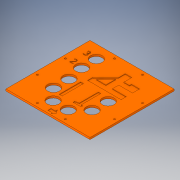
# Autodesk Inventor part: ControlPlateClimber
Saved by Autodesk Inventor 2019 (Build 230136000, 136)
## iProperties
Created: 2019-01-04
Part Number: ControlPlateClimber
Material: Generic
Document SubType Name: Modeling
Designer: james
Density: 1 g/cm^3
Appearance: Default(1)
Author: james
Autodesk Inventor part; units mm, degrees
ref_plane "YZ Plane" through (0, 0, 0) normal (1, 0, 0) x (0, 1, 0)
ref_plane "XZ Plane" through (0, 0, 0) normal (0, 1, 0) x (-1, 0, 0)
ref_plane "XY Plane" through (0, 0, 0) normal (0, 0, 1) x (1, 0, 0)
sketch "Sketch1" plane through (0, 0, 0) normal (0, 1, 0) x (-1, 0, 0)
  line L0 (148.429, 108.1825) -> (-80.171, 108.1825)
  line L1 (-80.171, 108.1825) -> (-80.171, -120.4175)
  line L2 (-80.171, -120.4175) -> (148.429, -120.4175)
  line L3 (148.429, -120.4175) -> (148.429, 108.1825)
  point P0 (0, 0)
  dimension "d0" = 228.6
  dimension "d1" = 228.6
  constraints: 8 end point, 2 parallel, 1 horizontal, 1 perpendicular
  measures "d0" distance of L0.end L1.end
  measures "d1" distance of L0.start L0.end
extrude "Extrusion1" add sketch "Sketch1" along normal blind 5.08
sketch "Sketch2" plane through (0, 5.08, 0) normal (0, 1, 0) x (1, 0, 0)
  line L0 (-148.429, -108.1825) -> (80.171, -108.1825) projected
  line L1 (80.171, 120.4175) -> (-148.429, 120.4175) projected
  line L2 (-148.429, 120.4175) -> (-148.429, -108.1825) projected
  line L3 (80.171, -108.1825) -> (80.171, 120.4175) projected
  point P0 (0, 0)
  point P1 (-138.904, -31.9825)
  point P2 (-138.904, 44.2175)
  point P3 (-72.229, 110.8925)
  point P4 (3.971, 110.8925)
  point P5 (70.646, 44.2175)
  point P6 (70.646, -31.9825)
  point P7 (-72.229, -98.6575)
  point P8 (3.971, -98.6575)
  dimension "d4" = 76.2
  dimension "d5" = 76.2
  dimension "d6" = 76.2
  dimension "d7" = 9.525
  dimension "d8" = 9.525
  dimension "d9" = 76.2
  dimension "d10" = 9.525
  dimension "d11" = 76.2
  dimension "d12" = 9.525
  dimension "d13" = 9.525
  measures "d4" distance from line of L0 point (-138.904, -31.983)
  measures "d5" distance of point (-138.904, 44.217) point (-138.904, -31.983)
  measures "d6" distance from line of L1 point (-138.904, 44.217)
  measures "d7" distance from line of L2 point (-138.904, 44.217)
  measures "d8" distance from line of L2 point (-138.904, -31.983)
  measures "d9" distance from line of point (-72.229, 110.892) L2
  measures "d10" distance from line of L1 point (-72.229, 110.892)
  measures "d11" distance of point (3.971, 110.892) point (-72.229, 110.892)
  measures "d12" distance from line of L3 point (70.646, 44.217)
  measures "d13" distance from line of L0 point (-72.229, -98.658)
hole "Hole1" at (-138.904, 5.08, 31.9825) at (-138.904, 5.08, -44.2175) at (-72.229, 5.08, -110.8925) at (3.971, 5.08, -110.8925) at (70.646, 5.08, -44.2175) at (70.646, 5.08, 31.9825) at (-72.229, 5.08, 98.6575) at (3.971, 5.08, 98.6575) direction (0, -1, 0) diameter 4.826 end through all
sketch "Sketch4" plane through (0, 5.08, 0) normal (0, 1, 0) x (1, 0, 0)
  line L0 (-57.5475, 37.222) -> (33.43, 37.222)
  line L1 (33.43, 37.222) -> (33.43, 23.0153)
  line L2 (33.43, 23.0153) -> (-57.5475, 23.0153)
  line L3 (-57.5475, 23.0153) -> (-57.5475, 37.222)
  line L4 (-22.0308, 37.222) -> (-3.9992, 37.222)
  line L5 (-3.9992, 37.222) -> (-3.9992, 89.9507)
  line L6 (-3.9992, 89.9507) -> (-22.0308, 89.9507)
  line L7 (-22.0308, 89.9507) -> (-22.0308, 37.222)
  line L8 (-22.0308, 71.0995) -> (-55.0887, 37.222)
  line L9 (-22.0308, 63.5863) -> (-47.7573, 37.222)
  line L10 (11.3003, 73.5584) -> (33.43, 73.5584)
  line L11 (33.43, 73.5584) -> (33.43, 54.1607)
  line L12 (33.43, 54.1607) -> (11.3003, 54.1607)
  line L13 (11.3003, 54.1607) -> (11.3003, 73.5584)
  line L14 (11.3003, 54.1607) -> (-3.9992, 54.1607)
  line L15 (11.3003, 68.0942) -> (-3.9992, 68.0942)
  point P0 (0, 0)
  constraints: 32 end point, 7 parallel, 7 point on line, 4 perpendicular, 3 horizontal, 1 midpoint
extrude "Extrusion2" cut sketch "Sketch4" against normal blind 1.651 contours L0 L1 L2 L3 | L8 L7 L9 L0 | L7 L6 L5 L0 | L5 L15 L13 L14 | L13 L10 L11 L12
sketch "Sketch5" plane through (0, 5.08, 0) normal (0, 1, 0) x (1, 0, 0)
  point P0 (0, 0)
  point P1 (-96.0634, 85.1626)
  point P2 (-95.5184, 44.5571)
  point P3 (19.7577, 1.7714)
  point P4 (18.6676, -41.0143)
  point P5 (-86.5252, 1.2263)
  point P6 (-86.5252, -40.7418)
  point P7 (-14.5798, -72.6266)
  point P8 (-56.8205, -71.5366)
hole "Hole2" at (-96.0634, 5.08, -85.1626) at (-95.5184, 5.08, -44.5571) at (19.7577, 5.08, -1.7714) at (18.6676, 5.08, 41.0143) at (-86.5252, 5.08, -1.2263) at (-86.5252, 5.08, 40.7418) at (-14.5798, 5.08, 72.6266) at (-56.8205, 5.08, 71.5366) direction (0, -1, 0) diameter 31.75 depth 25.4 tip angle 118.188
sketch "Sketch6" plane through (0, 5.08, 0) normal (0, 1, 0) x (1, 0, 0)
  line L0 (-63.361, 9.947) -> (-63.361, -48.3723)
  line L1 (-63.361, -48.3723) -> (-55.4579, -48.3723)
  line L2 (-55.4579, -48.3723) -> (-55.4579, 9.947)
  line L3 (-55.4579, 9.947) -> (-63.361, 9.947)
  line L4 (-15.3974, 9.947) -> (-8.5844, 9.947)
  line L5 (-8.5844, 9.947) -> (-8.5844, -43.467)
  line L6 (-8.5844, -43.467) -> (-3.9515, -43.467)
  line L7 (-3.9515, -43.467) -> (-3.9515, -48.3723)
  line L8 (-3.9515, -48.3723) -> (-25.7532, -48.3723)
  line L9 (-25.7532, -48.3723) -> (-25.7532, -43.467)
  line L10 (-25.7532, -43.467) -> (-15.3974, -42.1044)
  line L11 (-15.3974, -42.1044) -> (-15.3974, 9.947)
  line L12 (-41.1372, -92.7706) -> (-29.2067, -92.7706)
  line L13 (-29.2067, -92.7706) -> (-29.2067, -87.6575)
  line L14 (-29.2067, -87.6575) -> (-21.9024, -97.8836)
  line L15 (-21.9024, -97.8836) -> (-29.2067, -104.9445)
  line L16 (-29.2067, -104.9445) -> (-29.2067, -101.4141)
  line L17 (-29.2067, -101.4141) -> (-41.1372, -101.4141)
  line L18 (-41.1372, -101.4141) -> (-41.1372, -92.7706)
  point P0 (0, 0)
  constraints: 38 end point, 10 perpendicular, 7 point on line, 1 horizontal, 1 parallel, 1 vertical
extrude "Extrusion3" cut sketch "Sketch6" against normal blind 1.651
sketch "Sketch7" plane through (0, 5.08, 0) normal (0, 1, 0) x (1, 0, 0)
  line L0 (-127.4032, 94.1557) -> (-105.6016, 94.1557) construction
  line L1 (-105.6016, 94.1557) -> (-105.6016, 63.361) construction
  line L2 (-105.6016, 63.361) -> (-127.4032, 63.361) construction
  line L3 (-127.4032, 63.361) -> (-127.4032, 94.1557) construction
  spline S0 degree 2 poles (-122.1791, 92.3897) (-122.7349, 92.3897) (-123.834, 92.118) (-124.3651, 91.908) knots 0 0 0 1 2 2 2
  spline S1 degree 2 poles (-124.3651, 91.908) (-124.8591, 91.6981) (-125.5878, 91.2535) (-125.8718, 91.0559) knots 0 0 0 1 2 2 2
  line L4 (-125.8718, 91.0559) -> (-125.9953, 91.0559)
  line L5 (-125.9953, 91.0559) -> (-125.9953, 93.2171)
  spline S2 degree 2 poles (-125.9953, 93.2171) (-125.3284, 93.5753) (-123.0436, 94.1557) (-122.0186, 94.1557) knots 0 0 0 1 2 2 2
  spline S3 degree 2 poles (-122.0186, 94.1557) (-120.9812, 94.1557) (-119.4374, 93.7358) (-118.8076, 93.2912) knots 0 0 0 1 2 2 2
  spline S4 degree 2 poles (-118.8076, 93.2912) (-118.1407, 92.8096) (-117.4491, 91.414) (-117.4491, 90.4754) knots 0 0 0 1 2 2 2
  spline S5 degree 2 poles (-117.4491, 90.4754) (-117.4491, 89.2157) (-119.104, 87.3138) (-120.2649, 87.0668) knots 0 0 0 1 2 2 2
  line L6 (-120.2649, 87.0668) -> (-120.2649, 86.9186)
  spline S6 degree 2 poles (-120.2649, 86.9186) (-119.7832, 86.8198) (-118.6841, 86.3752) (-118.2148, 85.9306) knots 0 0 0 1 2 2 2
  spline S7 degree 2 poles (-118.2148, 85.9306) (-117.7455, 85.4983) (-117.1527, 84.1151) (-117.1527, 83.1148) knots 0 0 0 1 2 2 2
  spline S8 degree 2 poles (-117.1527, 83.1148) (-117.1527, 82.0897) (-117.8566, 80.3484) (-118.4988, 79.6815) knots 0 0 0 1 2 2 2
  spline S9 degree 2 poles (-118.4988, 79.6815) (-119.1657, 78.9898) (-121.0553, 78.2735) (-122.2532, 78.2735) knots 0 0 0 1 2 2 2
  spline S10 degree 2 poles (-122.2532, 78.2735) (-123.4018, 78.2735) (-125.6495, 78.8293) (-126.4152, 79.2121) knots 0 0 0 1 2 2 2
  line L7 (-126.4152, 79.2121) -> (-126.4152, 81.3734)
  line L8 (-126.4152, 81.3734) -> (-126.267, 81.3734)
  spline S11 degree 2 poles (-126.267, 81.3734) (-125.6248, 80.9041) (-123.4512, 80.0396) (-122.3767, 80.0396) knots 0 0 0 1 2 2 2
  spline S12 degree 2 poles (-122.3767, 80.0396) (-121.7469, 80.0396) (-120.4872, 80.4348) (-120.0673, 80.8918) knots 0 0 0 1 2 2 2
  spline S13 degree 2 poles (-120.0673, 80.8918) (-119.6597, 81.3487) (-119.2275, 82.4355) (-119.2275, 83.263) knots 0 0 0 1 2 2 2
  spline S14 degree 2 poles (-119.2275, 83.263) (-119.2275, 84.0904) (-119.7091, 85.1649) (-120.1414, 85.4736) knots 0 0 0 1 2 2 2
  spline S15 degree 2 poles (-120.1414, 85.4736) (-120.5736, 85.7824) (-121.7469, 86.017) (-122.4385, 86.017) knots 0 0 0 1 2 2 2
  line L9 (-122.4385, 86.017) -> (-123.303, 86.017)
  line L10 (-123.303, 86.017) -> (-123.303, 87.709)
  line L11 (-123.303, 87.709) -> (-122.6237, 87.709)
  spline S16 degree 2 poles (-122.6237, 87.709) (-121.2529, 87.709) (-119.5239, 89.0181) (-119.5239, 90.2655) knots 0 0 0 1 2 2 2
  spline S17 degree 2 poles (-119.5239, 90.2655) (-119.5239, 90.8459) (-119.9685, 91.6734) (-120.3266, 91.9204) knots 0 0 0 1 2 2 2
  spline S18 degree 2 poles (-120.3266, 91.9204) (-120.7095, 92.1797) (-121.6481, 92.3897) (-122.1791, 92.3897) knots 0 0 0 1 2 2 2
  point P0 (0, 0)
  constraints: 2 other
extrude "Extrusion4" cut sketch "Sketch7" against normal blind 1.651
sketch "Sketch8" plane through (0, 5.08, 0) normal (0, 1, 0) x (1, 0, 0)
  line L0 (-127.2171, 57.5261) -> (-116.4954, 57.5261) construction
  line L1 (-116.4954, 57.5261) -> (-116.4954, 35.2579) construction
  line L2 (-116.4954, 35.2579) -> (-127.2171, 35.2579) construction
  line L3 (-127.2171, 35.2579) -> (-127.2171, 57.5261) construction
  line L4 (-116.7072, 41.965) -> (-126.1056, 41.965)
  line L5 (-126.1056, 41.965) -> (-126.1056, 44.1262)
  spline S0 degree 2 poles (-126.1056, 44.1262) (-125.0929, 45.0772) (-123.2898, 46.8432) (-122.4253, 47.7942) knots 0 0 0 1 2 2 2
  spline S1 degree 2 poles (-122.4253, 47.7942) (-120.6839, 49.7085) (-119.4119, 52.0056) (-119.4119, 53.2282) knots 0 0 0 1 2 2 2
  spline S2 degree 2 poles (-119.4119, 53.2282) (-119.4119, 53.8704) (-119.8071, 54.8337) (-120.1652, 55.1425) knots 0 0 0 1 2 2 2
  spline S3 degree 2 poles (-120.1652, 55.1425) (-120.5234, 55.4512) (-121.462, 55.76) (-122.0301, 55.76) knots 0 0 0 1 2 2 2
  spline S4 degree 2 poles (-122.0301, 55.76) (-122.5735, 55.76) (-123.685, 55.4883) (-124.1913, 55.2783) knots 0 0 0 1 2 2 2
  spline S5 degree 2 poles (-124.1913, 55.2783) (-124.6236, 55.1054) (-125.4264, 54.6114) (-125.6734, 54.4385) knots 0 0 0 1 2 2 2
  line L6 (-125.6734, 54.4385) -> (-125.7845, 54.4385)
  line L7 (-125.7845, 54.4385) -> (-125.7845, 56.6122)
  spline S6 degree 2 poles (-125.7845, 56.6122) (-125.1547, 56.9209) (-122.8946, 57.5261) (-121.8819, 57.5261) knots 0 0 0 1 2 2 2
  spline S7 degree 2 poles (-121.8819, 57.5261) (-119.7453, 57.5261) (-117.3371, 55.266) (-117.3371, 53.3394) knots 0 0 0 1 2 2 2
  spline S8 degree 2 poles (-117.3371, 53.3394) (-117.3371, 52.4378) (-117.757, 50.9311) (-118.1275, 50.2889) knots 0 0 0 1 2 2 2
  spline S9 degree 2 poles (-118.1275, 50.2889) (-118.498, 49.622) (-119.5724, 48.3129) (-120.1652, 47.683) knots 0 0 0 1 2 2 2
  spline S10 degree 2 poles (-120.1652, 47.683) (-121.1285, 46.6333) (-123.4874, 44.3856) (-124.1913, 43.731) knots 0 0 0 1 2 2 2
  line L8 (-124.1913, 43.731) -> (-116.7072, 43.731)
  line L9 (-116.7072, 43.731) -> (-116.7072, 41.965)
  point P0 (0, 0)
  constraints: 2 other
extrude "Extrusion5" cut sketch "Sketch8" against normal blind 1.651
equation "\"d0\" = ControlPlateLength"
equation "\"d1\" = ControlPlateLength"
equation "\"d2\" = WallWidth"
equation "\"d7\" = ControlHoleBoltHoleMid"
equation "\"d8\" = ControlHoleBoltHoleMid"
equation "\"d10\" = ControlHoleBoltHoleMid"
equation "\"d12\" = ControlHoleBoltHoleMid"
equation "\"d13\" = ControlHoleBoltHoleMid"
equation "\"DSLength\" = 1371.6"
equation "\"DSWidth\" = 304.8"
equation "\"DCDeckHeight\" = 76.2"
equation "\"WallWidth\" = 5.08"
equation "\"EdgeAngle\" = 10deg"
equation "\"LengthCuts\" = 152.4"
equation "\"WidthCuts\" = 50.8"
equation "\"PartLength\" = 228.6"
equation "\"PartWidth\" = 152.4"
equation "\"BoltHoldDiam\" = 6.35"
equation "\"ControlPlateLength\" = 228.6"
equation "\"ControlPlateWidth\" = 228.6"
equation "\"ControlPlateShelfLength\" = 19.05"
equation "\"ControlHoleLength\" = 190.5"
equation "\"ControlHoleWidth\" = 190.5"
equation "\"ControlHoleFromSide\" = 63.5"
equation "\"ControlHoleBoltHoleMid\" = 9.525"
equation "\"DU1CHLength\" = 146.05"
equation "\"DU1CHWidth\" = 69.85"
equation "\"CPFromBack\" = 63.5"
equation "\"CPDeckHeight\" = 71.12"
equation "\"CPFromSide\" = 63.5"
equation "\"ControlPlateScrewLength\" = 76.2"
equation "\"DSBackHeight\" = 127"
equation "\"BackShelf\" = 25.4"
equation "\"MainAngle\" = 168.22deg"
equation "\"CPDWidthHole\" = 120.65"
equation "\"CPDLengthHole\" = 146.05"
equation "\"DownBackHeight\" = 130.7084"
body "Solid1"
